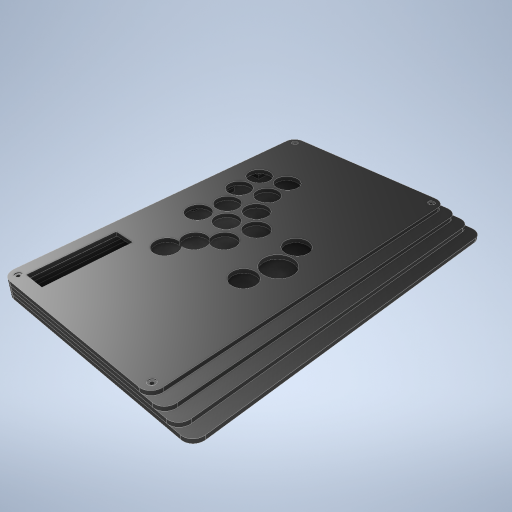
# Autodesk Inventor part: frame
Saved by Autodesk Inventor 2024 (Build 280153000, 153)
## iProperties
Created: 2023-10-17
Part Number: frame
Material: 玻璃
Document SubType Name: Modeling
Designer: Administrator
Density: 2.18 g/cm^3
Appearance: 有光泽 - 黑色
Author: Administrator
Autodesk Inventor part; units mm, degrees
ref_plane "YZ Plane" through (0, 0, 0) normal (1, 0, 0) x (0, 1, 0)
ref_plane "XY Plane" through (0, 0, 0) normal (0, 0, 1) x (1, 0, 0)
ref_plane "底层" through (0, -2, 0) normal (0, 1, 0) x (-1, 0, 0)
ref_plane "第二层" through (0, 4, 0) normal (0, 1, 0) x (-1, 0, 0)
ref_plane "第三层" through (0, 8, 0) normal (0, 1, 0) x (-1, 0, 0)
ref_plane "第四层" through (0, 12, 0) normal (0, 1, 0) x (-1, 0, 0)
sketch "第一层草图" plane through (0, 0, 0) normal (0, 1, 0) x (-1, 0, 0)
  line L0 (90, 150) -> (-90, 150)
  line L1 (-100, 140) -> (-100, -140)
  line L2 (-90, -150) -> (90, -150)
  line L3 (100, -140) -> (100, 140)
  line L4 (100, 150) -> (-100, -150) construction
  line L5 (-100, 150) -> (100, -150) construction
  arc A0 (100, 140) -> (90, 150) centre (90, 140) ccw
  arc A1 (-90, 150) -> (-100, 140) centre (-90, 140) ccw
  arc A2 (-100, -140) -> (-90, -150) centre (-90, -140) ccw
  arc A3 (90, -150) -> (100, -140) centre (90, -140) ccw
  point P0 (0, 0)
  dimension "d2" = 200
  dimension "d3" = 300
  dimension "d4" = 10
  constraints: 12 end point, 8 point on circle, 8 point on line, 8 tangent, 4 centre point, 3 equal radius, 2 midpoint, 2 parallel, 1 horizontal, 1 perpendicular
  measures "d2" distance of L5.end L4.end
  measures "d3" distance of L4.end L5.start
  measures "d4" radius of A0
sketch "第二层草图" plane through (0, 4, 0) normal (0, 1, 0) x (-1, 0, 0)
  line L0 (100, -140) -> (100, 140) projected
  line L1 (100, 0) -> (-88, 0)
  line L2 (90, 150) -> (-78, 150)
  line L3 (-88, 140) -> (-88, -140)
  line L4 (-78, -150) -> (90, -150)
  line L5 (100, -140) -> (100, 140)
  line L6 (100, 150) -> (-88, -150) construction
  line L7 (-88, 150) -> (100, -150) construction
  arc A0 (100, 140) -> (90, 150) centre (90, 140) ccw
  arc A1 (-78, 150) -> (-88, 140) centre (-78, 140) ccw
  arc A2 (-88, -140) -> (-78, -150) centre (-78, -140) ccw
  arc A3 (90, -150) -> (100, -140) centre (90, -140) ccw
  point P0 (0, 0)
  point P1 (6, 0)
  dimension "d101" = 188
  dimension "d102" = 188
  dimension "d103" = 300
  dimension "d104" = 10
  dimension "d125" = 10
  constraints: 14 end point, 8 point on circle, 8 point on line, 8 tangent, 4 centre point, 4 midpoint, 2 equal radius, 2 horizontal, 2 parallel, 1 perpendicular
  measures "d101" distance of L1.start L1.end
  measures "d102" distance of L7.end L6.end
  measures "d103" distance of L6.end L7.start
  measures "d104" radius of A0
  measures "d125" radius of A3
sketch "第三层草图" plane through (0, 8, 0) normal (0, 1, 0) x (-1, 0, 0)
  line L0 (100, -140) -> (100, 140) projected
  line L1 (100, 0) -> (-76, 0)
  line L2 (90, 150) -> (-66, 150)
  line L3 (-76, 140) -> (-76, -140)
  line L4 (-66, -150) -> (90, -150)
  line L5 (100, -140) -> (100, 140)
  line L6 (100, 150) -> (-76, -150) construction
  line L7 (-76, 150) -> (100, -150) construction
  arc A0 (100, 140) -> (90, 150) centre (90, 140) ccw
  arc A1 (-66, 150) -> (-76, 140) centre (-66, 140) ccw
  arc A2 (-76, -140) -> (-66, -150) centre (-66, -140) ccw
  arc A3 (90, -150) -> (100, -140) centre (90, -140) ccw
  point P0 (0, 0)
  point P1 (12, 0)
  dimension "d105" = 176
  dimension "d106" = 176
  dimension "d107" = 300
  dimension "d108" = 10
  constraints: 14 end point, 8 point on circle, 8 point on line, 8 tangent, 4 centre point, 4 midpoint, 3 equal radius, 2 horizontal, 2 parallel, 1 perpendicular
  measures "d105" distance of L1.start L1.end
  measures "d106" distance of L7.end L6.end
  measures "d107" distance of L6.end L7.start
  measures "d108" radius of A0
sketch "第四层草图" plane through (0, 12, 0) normal (0, 1, 0) x (-1, 0, 0)
  line L0 (100, -140) -> (100, 140) projected
  line L1 (100, 0) -> (-64, 0)
  line L2 (90, 150) -> (-54, 150)
  line L3 (-64, 140) -> (-64, -140)
  line L4 (-54, -150) -> (90, -150)
  line L5 (100, -140) -> (100, 140)
  line L6 (100, 150) -> (-64, -150) construction
  line L7 (-64, 150) -> (100, -150) construction
  arc A0 (100, 140) -> (90, 150) centre (90, 140) ccw
  arc A1 (-54, 150) -> (-64, 140) centre (-54, 140) ccw
  arc A2 (-64, -140) -> (-54, -150) centre (-54, -140) ccw
  arc A3 (90, -150) -> (100, -140) centre (90, -140) ccw
  point P0 (0, 0)
  point P1 (18, 0)
  dimension "d109" = 164
  dimension "d110" = 164
  dimension "d111" = 300
  dimension "d112" = 10
  dimension "d113" = 10
  constraints: 14 end point, 8 point on circle, 8 point on line, 8 tangent, 4 centre point, 4 midpoint, 2 equal radius, 2 horizontal, 2 parallel, 1 perpendicular
  measures "d109" distance of L1.start L1.end
  measures "d110" distance of L7.end L6.end
  measures "d111" distance of L6.end L7.start
  measures "d112" radius of A0
  measures "d113" radius of A2
sketch "底层草图" plane through (0, -2, 0) normal (0, 1, 0) x (-1, 0, 0)
  line L0 (98, 140) -> (98, -140)
  arc A0 (90, -148) -> (98, -140) centre (90, -140) ccw
  line L1 (90, -148) -> (-90, -148)
  arc A1 (-98, -140) -> (-90, -148) centre (-90, -140) ccw
  line L2 (-98, -140) -> (-98, 140)
  arc A2 (-90, 148) -> (-98, 140) centre (-90, 140) ccw
  line L3 (-90, 148) -> (90, 148)
  arc A3 (98, 140) -> (90, 148) centre (90, 140) ccw
  point P0 (0, 0)
  constraints: 8 end point, 8 point on circle, 4 centre point
extrude "拉伸25" add sketch "底层草图" along normal blind 2
extrude "拉伸26" add sketch "第一层草图" along normal blind 4 separate body
extrude "拉伸27" add sketch "第二层草图" along normal blind 4 separate body
extrude "拉伸28" add sketch "第三层草图" along normal blind 4 separate body
extrude "拉伸29" add sketch "第四层草图" along normal blind 4 separate body
sketch "草图20" plane through (0, 16, 0) normal (0, 1, 0) x (1, 0, 0)
  line L0 (-100, 140) -> (-100, -140) projected
  arc A0 (-100, -140) -> (-90, -150) centre (-90, -140) ccw projected
  line L1 (-90, -150) -> (54, -150) projected
  arc A1 (54, -150) -> (64, -140) centre (54, -140) ccw projected
  line L2 (64, -140) -> (64, 140) projected
  arc A2 (64, 140) -> (54, 150) centre (54, 140) ccw projected
  line L3 (54, 150) -> (-90, 150) projected
  arc A3 (-90, 150) -> (-100, 140) centre (-90, 140) ccw projected
  line L4 (-90, -140) -> (-92.1213, -142.1213)
  line L5 (-90, -140) -> (-87, -140) construction
  circle A4 centre (-92.1213, -142.1213) radius 2.75
  line L6 (-90, 140) -> (-92.1213, 142.1213)
  circle A5 centre (-92.1213, 142.1213) radius 2.75
  line L7 (54, -140) -> (56.1213, -142.1213)
  line L8 (54, -140) -> (57, -140) construction
  circle A6 centre (56.1213, -142.1213) radius 2.75
  line L9 (54, 140) -> (56.1213, 142.1213)
  circle A7 centre (56.1213, 142.1213) radius 2.75
  line L10 (-88, -138) -> (-88, 138)
  line L11 (-88, 138) -> (52, 138)
  line L12 (52, 138) -> (52, -138)
  line L13 (52, -138) -> (-88, -138)
  line L14 (-89.3713, -142.1213) -> (-90.7463, -144.5029)
  line L15 (-90.7463, -144.5029) -> (-93.4963, -144.5029)
  line L16 (-93.4963, -144.5029) -> (-94.8713, -142.1213)
  line L17 (-94.8713, -142.1213) -> (-93.4963, -139.7398)
  line L18 (-93.4963, -139.7398) -> (-90.7463, -139.7398)
  line L19 (-90.7463, -139.7398) -> (-89.3713, -142.1213)
  line L20 (-89.3713, 142.1213) -> (-90.7463, 139.7398)
  line L21 (-90.7463, 139.7398) -> (-93.4963, 139.7398)
  line L22 (-93.4963, 139.7398) -> (-94.8713, 142.1213)
  line L23 (-94.8713, 142.1213) -> (-93.4963, 144.5029)
  line L24 (-93.4963, 144.5029) -> (-90.7463, 144.5029)
  line L25 (-90.7463, 144.5029) -> (-89.3713, 142.1213)
  line L26 (58.8713, 142.1213) -> (57.4963, 139.7398)
  line L27 (57.4963, 139.7398) -> (54.7463, 139.7398)
  line L28 (54.7463, 139.7398) -> (53.3713, 142.1213)
  line L29 (53.3713, 142.1213) -> (54.7463, 144.5029)
  line L30 (54.7463, 144.5029) -> (57.4963, 144.5029)
  line L31 (57.4963, 144.5029) -> (58.8713, 142.1213)
  line L32 (58.8713, -142.1213) -> (57.4963, -144.5029)
  line L33 (57.4963, -144.5029) -> (54.7463, -144.5029)
  line L34 (54.7463, -144.5029) -> (53.3713, -142.1213)
  line L35 (53.3713, -142.1213) -> (54.7463, -139.7398)
  line L36 (54.7463, -139.7398) -> (57.4963, -139.7398)
  line L37 (57.4963, -139.7398) -> (58.8713, -142.1213)
  circle A8 centre (-92.1213, -142.1213) radius 1.6
  circle A9 centre (-92.1213, 142.1213) radius 1.6
  circle A10 centre (56.1213, -142.1213) radius 1.6
  circle A11 centre (56.1213, 142.1213) radius 1.6
  point P0 (0, 0)
  dimension "d128" = 5.5
  dimension "d130" = 5.5
  dimension "d132" = 5.5
  dimension "d134" = 5.5
  dimension "d126" = 3
  dimension "d127" = 135
  dimension "d129" = 3
  dimension "d131" = 45
  dimension "d133" = 3
  dimension "d135" = 12
  dimension "d136" = 3.2
  dimension "d137" = 3.2
  dimension "d138" = 3.2
  dimension "d139" = 3.2
  constraints: 68 end point, 12 coincident, 4 centre point, 4 horizontal alignment, 2 equal length, 2 horizontal, 63 other
  measures "d126" distance of L4.start L4.end
  measures "d127" angle of L4 L5
  measures "d129" distance of L6.start L6.end
  measures "d131" angle of L7 L8
  measures "d133" distance of L9.start L9.end
  measures "d135" distance between parallel lines of L0 L10
  measures "d136" diameter of A8
  measures "d137" diameter of A9
  measures "d138" diameter of A10
  measures "d139" diameter of A11
extrude "拉伸30" cut sketch "草图20" against normal up to surface (18 mm away) contours L10 L11 L12 L13 bodies 4 3 2
hole "四角固定孔" at (-92.1213, 16, 142.1213) at (-92.1213, 16, -142.1213) at (56.1213, 16, -142.1213) at (56.1213, 16, 142.1213) direction (0, -1, 0) diameter 3.2 end through all counterbore diameter 6.2 counterbore depth 1 bodies 5
extrude "六角通孔1" cut sketch "草图20" against normal through all contours L19 L14 L15 L16 L17 L18 | A8 bodies 4 3 2
extrude "六角通孔2" cut sketch "草图20" against normal through all contours L35 L36 L37 L32 L33 L34 | A10 bodies 4 3 2
extrude "六角通孔3" cut sketch "草图20" against normal through all contours L28 L29 L30 L31 L26 L27 | A11 bodies 4 3 2
extrude "六角通孔4" cut sketch "草图20" against normal through all contours L20 L21 L22 L23 L24 L25 | A9 bodies 4 3 2
sketch "第二层开孔草图" plane through (0, 8, 0) normal (0, 1, 0) x (1, 0, 0)
  line L0 (-100, 0) -> (-98, 0)
  line L1 (-100, 0) -> (-98, 0) construction
  line L2 (-98, 0) -> (-88, 0)
  line L3 (-98, -15) -> (-88, -15)
  line L4 (-88, -15) -> (-88, 15)
  line L5 (-88, 15) -> (-98, 15)
  line L6 (-98, 15) -> (-98, -15)
  line L7 (-98, -15) -> (-88, 15) construction
  line L8 (-88, -15) -> (-98, 15) construction
  line L9 (-100, -4.9) -> (-98, -4.9)
  line L10 (-98, -4.9) -> (-98, 4.9)
  line L11 (-98, 4.9) -> (-100, 4.9)
  line L12 (-100, 4.9) -> (-100, -4.9)
  line L13 (-100, -4.9) -> (-98, 4.9) construction
  line L14 (-98, -4.9) -> (-100, 4.9) construction
  line L15 (-88, 76.5) -> (-98, 76.5)
  line L16 (-98, 76.5) -> (-100, 76.5)
  line L17 (-98, 76.5) -> (-96, 76.5) construction
  line L18 (-98, 61.5) -> (-88, 61.5)
  line L19 (-88, 61.5) -> (-88, 91.5)
  line L20 (-88, 91.5) -> (-98, 91.5)
  line L21 (-98, 91.5) -> (-98, 61.5)
  line L22 (-98, 61.5) -> (-88, 91.5) construction
  line L23 (-88, 61.5) -> (-98, 91.5) construction
  line L24 (-100, 71.6) -> (-98, 71.6)
  line L25 (-98, 71.6) -> (-98, 81.4)
  line L26 (-98, 81.4) -> (-100, 81.4)
  line L27 (-100, 81.4) -> (-100, 71.6)
  line L28 (-100, 71.6) -> (-98, 81.4) construction
  line L29 (-98, 71.6) -> (-100, 81.4) construction
  line L30 (-88, 15) -> (-88, 61.5)
  line L31 (-88, 38.25) -> (-100, 38.25)
  line L32 (-100, 26.75) -> (-88, 26.75)
  line L33 (-88, 26.75) -> (-88, 49.75)
  line L34 (-88, 49.75) -> (-100, 49.75)
  line L35 (-100, 49.75) -> (-100, 26.75)
  line L36 (-100, 26.75) -> (-88, 49.75) construction
  line L37 (-88, 26.75) -> (-100, 49.75) construction
  line L38 (-91.2527, 26.75) -> (-92.6263, 24.3708)
  line L39 (-92.6263, 24.3708) -> (-95.3737, 24.3708)
  line L40 (-95.3737, 24.3708) -> (-96.7473, 26.75)
  line L41 (-96.7473, 26.75) -> (-95.3737, 29.1292)
  line L42 (-95.3737, 29.1292) -> (-92.6263, 29.1292)
  line L43 (-92.6263, 29.1292) -> (-91.2527, 26.75)
  line L44 (-91.2527, 49.75) -> (-92.6263, 47.3708)
  line L45 (-92.6263, 47.3708) -> (-95.3737, 47.3708)
  line L46 (-95.3737, 47.3708) -> (-96.7473, 49.75)
  line L47 (-96.7473, 49.75) -> (-95.3737, 52.1292)
  line L48 (-95.3737, 52.1292) -> (-92.6263, 52.1292)
  line L49 (-92.6263, 52.1292) -> (-91.2527, 49.75)
  line L50 (-88, -15) -> (-88, -26.75)
  line L51 (-88, -26.75) -> (-100, -26.75)
  line L52 (-88, 91.5) -> (-88, 103.25)
  line L53 (-88, 103.25) -> (-100, 103.25)
  line L54 (-91.2501, -26.75) -> (-92.625, -29.1315)
  line L55 (-92.625, -29.1315) -> (-95.375, -29.1315)
  line L56 (-95.375, -29.1315) -> (-96.7499, -26.75)
  line L57 (-96.7499, -26.75) -> (-95.375, -24.3685)
  line L58 (-95.375, -24.3685) -> (-92.625, -24.3685)
  line L59 (-92.625, -24.3685) -> (-91.2501, -26.75)
  line L60 (-91.2501, 103.25) -> (-92.625, 100.8685)
  line L61 (-92.625, 100.8685) -> (-95.375, 100.8685)
  line L62 (-95.375, 100.8685) -> (-96.7499, 103.25)
  line L63 (-96.7499, 103.25) -> (-95.375, 105.6315)
  line L64 (-95.375, 105.6315) -> (-92.625, 105.6315)
  line L65 (-92.625, 105.6315) -> (-91.2501, 103.25)
  point P0 (0, 0)
  point P1 (-93, 0)
  point P2 (-99, 0)
  point P3 (-93, 76.5)
  point P4 (-99, 76.5)
  point P5 (-94, 38.25)
  point P6 (-94, 26.75)
  point P7 (-94, 49.75)
  point P8 (-94, -26.75)
  point P9 (-94, 103.25)
  dimension "d164" = 2
  dimension "d165" = 0
  dimension "d166" = 30
  dimension "d167" = 9.8
  dimension "d172" = 10
  dimension "d173" = 2
  dimension "d174" = 180
  dimension "d175" = 10
  dimension "d176" = 30
  dimension "d177" = 2
  dimension "d178" = 9.8
  dimension "d183" = 23
  dimension "d189" = 11.75
  dimension "d190" = 11.75
  constraints: 132 end point, 10 midpoint, 2 collinear, 2 horizontal, 52 other
  measures "d164" distance of L0.start L0.end
  measures "d165" distance between parallel lines of L0 L1
  measures "d166" distance of L4.end L3.end
  measures "d167" distance of L10.end L9.end
  measures "d172" distance of L15.start L15.end
  measures "d173" distance of L16.start L16.end
  measures "d174" angle of L16 L17
  measures "d175" distance of L20.end L19.end
  measures "d176" distance of L19.end L18.end
  measures "d177" distance of L26.end L25.end
  measures "d178" distance of L25.end L24.end
  measures "d183" distance of L33.end L32.end
  measures "d189" distance of L50.start L50.end
  measures "d190" distance of L52.start L52.end
extrude "拉伸35" cut sketch "第二层开孔草图" against normal blind 10 contours L6 L5 L4 L2 | L2 L4 L3 L6 bodies 3 2
extrude "拉伸36" cut sketch "第二层开孔草图" against normal blind 10 contours L12 L11 L6 L0 | L0 L6 L9 L12 bodies 3
extrude "拉伸37" cut sketch "第二层开孔草图" against normal through all contours L19 L18 L21 L15 | L15 L21 L20 L19 bodies 3 2
extrude "拉伸38" cut sketch "第二层开孔草图" against normal through all contours L21 L24 L27 L16 | L16 L27 L26 L21 bodies 3
ref_plane "第三层开孔面" through (0, 12, 0) normal (0, 1, 0) x (1, 0, 0)
sketch "第三层开孔草图" plane through (0, 12, 0) normal (0, 1, 0) x (1, 0, 0)
  line L0 (-95.3737, 29.1292) -> (-92.6263, 29.1292) projected
  line L1 (-96.7473, 26.75) -> (-95.3737, 29.1292) projected
  line L2 (-95.3737, 24.3708) -> (-96.7473, 26.75) projected
  line L3 (-92.6263, 24.3708) -> (-95.3737, 24.3708) projected
  line L4 (-91.2527, 26.75) -> (-92.6263, 24.3708) projected
  line L5 (-92.6263, 29.1292) -> (-91.2527, 26.75) projected
  line L6 (-91.2527, 49.75) -> (-92.6263, 47.3708) projected
  line L7 (-92.6263, 47.3708) -> (-95.3737, 47.3708) projected
  line L8 (-95.3737, 47.3708) -> (-96.7473, 49.75) projected
  line L9 (-96.7473, 49.75) -> (-95.3737, 52.1292) projected
  line L10 (-95.3737, 52.1292) -> (-92.6263, 52.1292) projected
  line L11 (-92.6263, 52.1292) -> (-91.2527, 49.75) projected
  line L12 (-96.7499, -26.75) -> (-95.375, -24.3685) projected
  line L13 (-95.375, -29.1315) -> (-96.7499, -26.75) projected
  line L14 (-92.625, -29.1315) -> (-95.375, -29.1315) projected
  line L15 (-91.2501, -26.75) -> (-92.625, -29.1315) projected
  line L16 (-92.625, -24.3685) -> (-91.2501, -26.75) projected
  line L17 (-95.375, -24.3685) -> (-92.625, -24.3685) projected
  line L18 (-95.375, 100.8685) -> (-96.7499, 103.25) projected
  line L19 (-92.625, 100.8685) -> (-95.375, 100.8685) projected
  line L20 (-91.2501, 103.25) -> (-92.625, 100.8685) projected
  line L21 (-92.625, 105.6315) -> (-91.2501, 103.25) projected
  line L22 (-95.375, 105.6315) -> (-92.625, 105.6315) projected
  line L23 (-96.7499, 103.25) -> (-95.375, 105.6315) projected
  point P0 (0, 0)
extrude "中间层固定孔" cut sketch "第三层开孔草图" against normal through all bodies 4 3 2
sketch "底部孔草图" plane through (0, -2, 0) normal (0, -1, 0) x (1, 0, 0)
  circle A0 centre (-92.1213, -142.1213) radius 2.75 projected
  circle A1 centre (56.1213, -142.1213) radius 2.75 projected
  circle A2 centre (56.1213, 142.1213) radius 2.75 projected
  circle A3 centre (-92.1213, 142.1213) radius 2.75 projected
  line L0 (-96.7473, -26.75) -> (-95.3737, -24.3708) projected
  line L1 (-95.3737, -29.1292) -> (-96.7473, -26.75) projected
  line L2 (-92.6263, -29.1292) -> (-95.3737, -29.1292) projected
  line L3 (-91.2527, -26.75) -> (-92.6263, -29.1292) projected
  line L4 (-92.6263, -24.3708) -> (-91.2527, -26.75) projected
  line L5 (-95.3737, -24.3708) -> (-92.6263, -24.3708) projected
  line L6 (-95.375, 24.3685) -> (-96.7499, 26.75) projected
  line L7 (-96.7499, 26.75) -> (-95.375, 29.1315) projected
  line L8 (-95.375, 29.1315) -> (-92.625, 29.1315) projected
  line L9 (-92.625, 29.1315) -> (-91.2501, 26.75) projected
  line L10 (-91.2501, 26.75) -> (-92.625, 24.3685) projected
  line L11 (-92.625, 24.3685) -> (-95.375, 24.3685) projected
  circle A4 centre (-94, -26.75) radius 2.3792
  circle A5 centre (-94, 26.75) radius 2.3815
  point P0 (0, 0)
  constraints: 6 tangent, 2 centre point
hole "底板定位孔" at (-92.1213, -2, -142.1213) at (-92.1213, -2, 142.1213) at (56.1213, -2, 142.1213) at (56.1213, -2, -142.1213) at (-94, -2, -26.75) at (-94, -2, 26.75) direction (0, 1, 0) diameter 3.2 end through all counterbore diameter 6.2 counterbore depth 1 bodies 1
ref_plane "按键孔位平面" through (0, 16, 0) normal (0, 1, 0) x (1, 0, 0)
sketch "按键孔位图" plane through (0, 16, 0) normal (0, 1, 0) x (1, 0, 0)
  circle A0 centre (-65.0378, 1.142) radius 11.5
  circle A1 centre (-58.3085, 26.2561) radius 11.5
  circle A2 centre (-39.9237, 7.8713) radius 11.5
  line L0 (-39.9237, 7.8713) -> (-39.9237, 33.8713)
  line L1 (-21.2884, -11.7513) -> (-21.2884, 10.2487)
  line L2 (-39.9237, 7.8713) -> (-58.3085, 26.2561)
  line L3 (-58.3085, 26.2561) -> (-69.2965, 49.8201)
  line L4 (-69.2965, 49.8201) -> (-71.5626, 75.7211)
  line L5 (-21.2884, -11.7513) -> (-36.8447, -27.3076)
  line L6 (-36.8447, -27.3076) -> (-46.1423, -47.2464)
  circle A3 centre (-36.8447, -27.3076) radius 11.5
  line L7 (-15.2859, 15.7913) -> (-33.6707, 34.176)
  line L8 (-33.6707, 34.176) -> (-44.6587, 57.74)
  line L9 (-44.6587, 57.74) -> (-46.9248, 83.6411)
  circle A4 centre (-21.2884, -11.7513) radius 11.5
  circle A5 centre (-69.2965, 49.8201) radius 11.5
  circle A6 centre (-33.6707, 34.176) radius 11.5
  line L10 (-15.2859, 15.7913) -> (-15.2859, 41.7913)
  circle A7 centre (-15.2859, 15.7913) radius 11.5
  circle A8 centre (-46.1423, -47.2464) radius 11.5
  circle A9 centre (-44.6587, 57.74) radius 11.5
  circle A10 centre (-71.5626, 75.7211) radius 11.5
  circle A11 centre (-46.9248, 83.6411) radius 11.5
  circle A12 centre (21.9427, 20.1213) radius 11.5
  circle A13 centre (21.9427, -33.997) radius 11.5
  circle A14 centre (29.1401, -6.9379) radius 14.5
  line L11 (-88, -138) -> (-88, -128)
  line L12 (-88, -128) -> (-78, -128)
  line L13 (-88, -128) -> (-78, -128) construction
  line L14 (-68.85, -137.15) -> (-68.85, -118.85)
  line L15 (-68.85, -118.85) -> (-87.15, -118.85)
  line L16 (-87.15, -118.85) -> (-87.15, -137.15)
  line L17 (-87.15, -137.15) -> (-68.85, -118.85) construction
  line L18 (-68.85, -137.15) -> (-87.15, -118.85) construction
  line L19 (-78, -128) -> (-78, -109)
  line L20 (-78, -128) -> (-59, -128) construction
  line L21 (-78, -109) -> (-78, -90)
  line L22 (-78, -90) -> (-78, -71)
  line L23 (-87.15, -118.15) -> (-68.85, -118.15)
  line L24 (-68.85, -118.15) -> (-68.85, -99.85)
  line L25 (-68.85, -99.85) -> (-87.15, -99.85)
  line L26 (-87.15, -99.85) -> (-87.15, -118.15)
  line L27 (-87.15, -118.15) -> (-68.85, -99.85) construction
  line L28 (-68.85, -118.15) -> (-87.15, -99.85) construction
  line L29 (-87.15, -99.15) -> (-68.85, -99.15)
  line L30 (-68.85, -99.15) -> (-68.85, -80.85)
  line L31 (-68.85, -80.85) -> (-87.15, -80.85)
  line L32 (-87.15, -80.85) -> (-87.15, -99.15)
  line L33 (-87.15, -99.15) -> (-68.85, -80.85) construction
  line L34 (-68.85, -99.15) -> (-87.15, -80.85) construction
  line L35 (-87.15, -80.15) -> (-68.85, -80.15)
  line L36 (-68.85, -80.15) -> (-68.85, -61.85)
  line L37 (-87.15, -61.85) -> (-87.15, -80.15)
  line L38 (-87.15, -80.15) -> (-68.85, -61.85) construction
  line L39 (-68.85, -80.15) -> (-87.15, -61.85) construction
  line L40 (-87.15, -137.15) -> (-68.85, -137.15)
  line L41 (-68.85, -61.85) -> (-87.15, -61.85)
  line L42 (-67.85, -60.85) -> (-67.85, -138.15)
  line L43 (-67.85, -138.15) -> (-88.15, -138.15)
  line L44 (-88.15, -138.15) -> (-88.15, -60.85)
  line L45 (-88.15, -60.85) -> (-67.85, -60.85)
  point P0 (0, 0)
  point P1 (-44.5334, -35.8595)
  point P2 (-38.4537, -38.6945)
  point P3 (-26.6948, -21.9012)
  point P4 (-31.4383, -17.1578)
  dimension "d195" = 10
  dimension "d196" = 10
  dimension "d197" = 0
  dimension "d198" = 18.3
  dimension "d199" = 18.3
  dimension "d200" = 19
  dimension "d201" = 90
  dimension "d202" = 19
  dimension "d203" = 19
  dimension "d204" = 18.3
  dimension "d205" = 18.3
  dimension "d206" = 18.3
  dimension "d207" = 18.3
  dimension "d208" = 18.3
  dimension "d209" = 18.3
  constraints: 92 end point, 15 centre point, 8 midpoint, 2 equal length, 2 horizontal
  measures "d195" distance of L11.start L11.end
  measures "d196" distance of L12.start L12.end
  measures "d197" distance between parallel lines of L12 L13
  measures "d198" distance of L15.end L14.end
  measures "d199" distance of L14.end L14.start
  measures "d200" distance of L19.start L19.end
  measures "d201" angle of L20 L19
  measures "d202" distance of L21.start L21.end
  measures "d203" distance of L22.start L22.end
  measures "d204" distance of L25.end L24.end
  measures "d205" distance of L24.end L23.end
  measures "d206" distance of L31.end L30.end
  measures "d207" distance of L30.end L29.end
  measures "d208" distance of L37.start L36.end
  measures "d209" distance of L36.end L35.end
extrude "按键开孔" cut sketch "按键孔位图" against normal through all contours A0 | A1 L2 L3 | L3 L2 A1 | A2 L2 L0 | L0 L2 A2 | L5 A3 A4 L1 | L1 A4 A3 L5 | A3 A4 L5 | L5 A4 A3 | A4 L5 L6 A8 A3 | A4 A3 A8 L6 L5 | A8 L6 A3 | A3 A8 | L6 A8 A3 | A5 L4 L3 | L3 L4 A5 | L10 A7 L7 | L7 A7 L10 | A6 L8 L7 | L7 L8 A6 | A9 L9 L8 | L8 L9 A9 | A10 | A11 | A12 | A13 | A14 | L16 L15 L19 L12 | L12 L19 L15 L14 L40 L16 | L23 L26 L25 L21 L19 | L19 L21 L25 L24 L23 | L29 L32 L31 L22 L21 | L21 L22 L31 L30 L29 | L37 L41 L36 L35 | L42 L43 L44 L45 bodies 5
